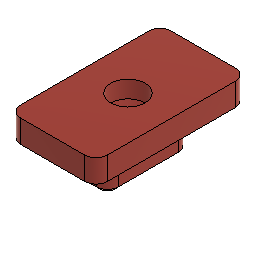
MEUBLE FAL_prod_BS (Autodesk Fusion 360 archive; units mm, degrees)
design "BLOCKOR_L36"
Autodesk Fusion 360 part; units mm, degrees
sketch "Sketch1" plane through (0, 0, 0) normal (0, 0, 1) x (1, 0, 0)
  line L0 (9, 18) -> (-9, 18)
  line L1 (-9, 18) -> (-9, -18)
  line L2 (-9, -18) -> (9, -18)
  line L3 (9, -18) -> (9, 18)
  line L4 (9, 18) -> (-9, -18) construction
  line L5 (-9, 18) -> (9, -18) construction
  dimension "d1" = 18
  dimension "d2" = 36
  constraint horizontal L0
  constraint perpendicular L0 L1
  constraint parallel L0 L2
  constraint parallel L1 L3
  constraint coincident L4 origin
  constraint coincident L5 origin
  measures "d1" distance of L0.start L0.end
  measures "d2" distance of L0.end L1.end
extrude "Extrude1" add sketch "Sketch1" along normal blind 16.5
sketch "Sketch2" plane through (0, 0, 16.5) normal (0, 0, 1) x (-1, 0, 0)
  line L0 (-9, 18) -> (-9, -18)
  line L1 (-9, -18) -> (9, -18)
  line L2 (9, -18) -> (9, 18)
  line L3 (9, 18) -> (-9, 18)
  line L4 (-19, -33) -> (19, -33)
  line L5 (19, -33) -> (19, 33)
  line L6 (19, 33) -> (-19, 33)
  line L7 (-19, 33) -> (-19, -33)
  line L8 (-19, -33) -> (19, 33) construction
  line L9 (19, -33) -> (-19, 33) construction
  dimension "d5" = 10
  dimension "d6" = 15
  constraint horizontal L4
  constraint perpendicular L4 L5
  constraint parallel L4 L6
  constraint parallel L5 L7
  constraint coincident L8 origin
  constraint coincident L9 origin
  measures "d5" distance of L2 L5
  measures "d6" distance of L1 L4
extrude "Extrude2" add sketch "Sketch2" along normal blind 10 contours L0 L1 L2 L3 | L4 L5 L6 L7
sketch "Sketch3" plane through (0, 0, 26.5) normal (0, 0, 1) x (-1, 0, 0)
  line L0 (-19, 33) -> (-19, -33)
  line L1 (-19, -33) -> (19, -33)
  line L2 (19, -33) -> (19, 33)
  line L3 (19, 33) -> (-19, 33)
  circle A0 centre (0, 0) radius 7.5
  dimension "d17" = 15
  constraint coincident A0.centre origin
  measures "d17" diameter of A0
extrude "Extrude3" cut sketch "Sketch3" against normal up to surface (10 mm away) contours A0
sketch "Sketch4" plane through (0, 0, 16.5) normal (0, 0, 1) x (-1, 0, 0)
  circle A0 centre (0, 0) radius 7.5
  constraint coincident A0.centre origin
hole "Hole2" at (0, 0, 16.5) direction (0, 0, -1) diameter 4.5 end through all countersink diameter 10 countersink angle 90
chamfer "Chamfer2" distance 2.5 angle 45 1 edges at (6.9925, 2.7121, 16.5)
fillet "Fillet1" radius 5 4 edges at (9, -18, 8.25) (-9, -18, 8.25) (9, 18, 8.25) (-9, 18, 8.25)
fillet "Fillet2" radius 5 4 edges at (-19, 33, 21.5) (19, 33, 21.5) (-19, -33, 21.5) (19, -33, 21.5)
chamfer "Chamfer1" distance 2 angle 45 8 edges at (0, 18, 0) (-7.5355, 16.5355, 0) (-9, 0, 0) (-7.5355, -16.5355, 0) (0, -18, 0) (7.5355, -16.5355, 0) (9, 0, 0) (7.5355, 16.5355, 0)

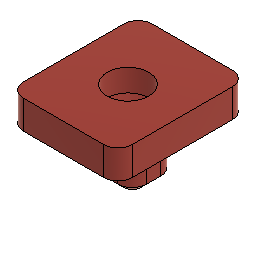
design "BLOCKOR_L15"
Autodesk Fusion 360 part; units mm, degrees
sketch "Sketch1" plane through (0, 0, 0) normal (0, 0, 1) x (1, 0, 0)
  line L0 (9, 7.5) -> (-9, 7.5)
  line L1 (-9, 7.5) -> (-9, -7.5)
  line L2 (-9, -7.5) -> (9, -7.5)
  line L3 (9, -7.5) -> (9, 7.5)
  line L4 (9, 7.5) -> (-9, -7.5) construction
  line L5 (-9, 7.5) -> (9, -7.5) construction
  dimension "d1" = 18
  dimension "d2" = 15
  constraint horizontal L0
  constraint perpendicular L0 L1
  constraint parallel L0 L2
  constraint parallel L1 L3
  constraint coincident L4 origin
  constraint coincident L5 origin
  measures "d1" distance of L0.start L0.end
  measures "d2" distance of L0.end L1.end
extrude "Extrude1" add sketch "Sketch1" along normal blind 16.5
sketch "Sketch2" plane through (0, 0, 16.5) normal (0, 0, 1) x (-1, 0, 0)
  line L0 (-9, 7.5) -> (-9, -7.5)
  line L1 (-9, -7.5) -> (9, -7.5)
  line L2 (9, -7.5) -> (9, 7.5)
  line L3 (9, 7.5) -> (-9, 7.5)
  line L4 (-19, -22.5) -> (19, -22.5)
  line L5 (19, -22.5) -> (19, 22.5)
  line L6 (19, 22.5) -> (-19, 22.5)
  line L7 (-19, 22.5) -> (-19, -22.5)
  line L8 (-19, -22.5) -> (19, 22.5) construction
  line L9 (19, -22.5) -> (-19, 22.5) construction
  dimension "d5" = 10
  dimension "d6" = 15
  constraint horizontal L4
  constraint perpendicular L4 L5
  constraint parallel L4 L6
  constraint parallel L5 L7
  constraint coincident L8 origin
  constraint coincident L9 origin
  measures "d5" distance of L2 L5
  measures "d6" distance of L1 L4
extrude "Extrude2" add sketch "Sketch2" along normal blind 10 contours L0 L1 L2 L3 | L4 L5 L6 L7
sketch "Sketch3" plane through (0, 0, 26.5) normal (0, 0, 1) x (-1, 0, 0)
  line L0 (-19, 22.5) -> (-19, -22.5)
  line L1 (-19, -22.5) -> (19, -22.5)
  line L2 (19, -22.5) -> (19, 22.5)
  line L3 (19, 22.5) -> (-19, 22.5)
  circle A0 centre (0, 0) radius 7.25
  dimension "d17" = 14.5
  constraint coincident A0.centre origin
  measures "d17" diameter of A0
fillet "Fillet1" radius 5 4 edges at (9, -7.5, 8.25) (-9, -7.5, 8.25) (9, 7.5, 8.25) (-9, 7.5, 8.25)
fillet "Fillet2" radius 5 4 edges at (-19, 22.5, 21.5) (19, 22.5, 21.5) (-19, -22.5, 21.5) (19, -22.5, 21.5)
chamfer "Chamfer1" distance 2 angle 45 8 edges at (0, 7.5, 0) (-7.5355, 6.0355, 0) (-9, 0, 0) (-7.5355, -6.0355, 0) (0, -7.5, 0) (7.5355, -6.0355, 0) (9, 0, 0) (7.5355, 6.0355, 0)
extrude "Extrude3" cut sketch "Sketch3" against normal up to surface (10 mm away) contours A0
sketch "Sketch4" plane through (0, 0, 16.5) normal (0, 0, 1) x (-1, 0, 0)
  circle A0 centre (0, 0) radius 7.25
  constraint coincident A0.centre origin
hole "Hole2" at (0, 0, 16.5) direction (0, 0, -1) diameter 4.5 end through all countersink diameter 10 countersink angle 90
chamfer "Chamfer2" distance 2.25 angle 45 1 edges at (6.7594, 2.6217, 16.5)

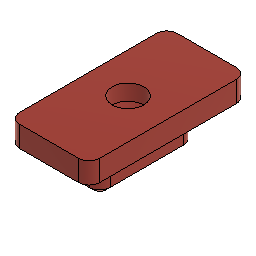
design "BLOCKOR_L45"
Autodesk Fusion 360 part; units mm, degrees
sketch "Sketch1" plane through (0, 0, 0) normal (0, 0, 1) x (1, 0, 0)
  line L0 (9, 22.5) -> (-9, 22.5)
  line L1 (-9, 22.5) -> (-9, -22.5)
  line L2 (-9, -22.5) -> (9, -22.5)
  line L3 (9, -22.5) -> (9, 22.5)
  line L4 (9, 22.5) -> (-9, -22.5) construction
  line L5 (-9, 22.5) -> (9, -22.5) construction
  dimension "d1" = 18
  dimension "d2" = 45
  constraint horizontal L0
  constraint perpendicular L0 L1
  constraint parallel L0 L2
  constraint parallel L1 L3
  constraint coincident L4 origin
  constraint coincident L5 origin
  measures "d1" distance of L0.start L0.end
  measures "d2" distance of L0.end L1.end
  measures "d5" distance of L0.start
  measures "d6" distance of L0.start
extrude "Extrude1" add sketch "Sketch1" along normal blind 16.5
sketch "Sketch2" plane through (0, 0, 16.5) normal (0, 0, 1) x (-1, 0, 0)
  line L0 (-9, 22.5) -> (-9, -22.5)
  line L1 (-9, -22.5) -> (9, -22.5)
  line L2 (9, -22.5) -> (9, 22.5)
  line L3 (9, 22.5) -> (-9, 22.5)
  line L4 (-19, -37.5) -> (19, -37.5)
  line L5 (19, -37.5) -> (19, 37.5)
  line L6 (19, 37.5) -> (-19, 37.5)
  line L7 (-19, 37.5) -> (-19, -37.5)
  line L8 (-19, -37.5) -> (19, 37.5) construction
  line L9 (19, -37.5) -> (-19, 37.5) construction
  dimension "d5" = 10
  dimension "d6" = 15
  constraint horizontal L4
  constraint perpendicular L4 L5
  constraint parallel L4 L6
  constraint parallel L5 L7
  constraint coincident L8 origin
  constraint coincident L9 origin
  measures "d5" distance of L2 L5
  measures "d6" distance of L1 L4
extrude "Extrude2" add sketch "Sketch2" along normal blind 10 contours L0 L1 L2 L3 | L4 L5 L6 L7
sketch "Sketch3" plane through (0, 0, 26.5) normal (0, 0, 1) x (-1, 0, 0)
  line L0 (-19, 37.5) -> (-19, -37.5)
  line L1 (-19, -37.5) -> (19, -37.5)
  line L2 (19, -37.5) -> (19, 37.5)
  line L3 (19, 37.5) -> (-19, 37.5)
  circle A0 centre (0, 0) radius 7.5
  dimension "d17" = 15
  constraint coincident A0.centre origin
  measures "d17" diameter of A0
extrude "Extrude3" cut sketch "Sketch3" against normal up to surface (10 mm away) contours A0
sketch "Sketch4" plane through (0, 0, 16.5) normal (0, 0, 1) x (-1, 0, 0)
  circle A0 centre (0, 0) radius 7.5
  constraint coincident A0.centre origin
hole "Hole2" at (0, 0, 16.5) direction (0, 0, -1) diameter 4.5 end through all countersink diameter 10 countersink angle 90
chamfer "Chamfer2" distance 2.5 angle 45 1 edges at (6.9925, 2.7121, 16.5)
fillet "Fillet1" radius 5 4 edges at (9, -22.5, 8.25) (-9, -22.5, 8.25) (9, 22.5, 8.25) (-9, 22.5, 8.25)
fillet "Fillet2" radius 5 4 edges at (-19, 37.5, 21.5) (19, 37.5, 21.5) (-19, -37.5, 21.5) (19, -37.5, 21.5)
chamfer "Chamfer1" distance 2 angle 45 8 edges at (0, 22.5, 0) (-7.5355, 21.0355, 0) (-9, 0, 0) (-7.5355, -21.0355, 0) (0, -22.5, 0) (7.5355, -21.0355, 0) (9, 0, 0) (7.5355, 21.0355, 0)

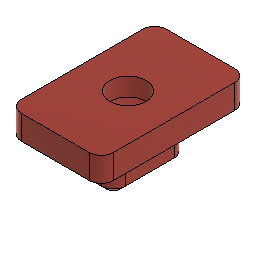
design "BLOCKOR_L30"
Autodesk Fusion 360 part; units mm, degrees
sketch "Sketch1" plane through (0, 0, 0) normal (0, 0, 1) x (1, 0, 0)
  line L0 (9, 15) -> (-9, 15)
  line L1 (-9, 15) -> (-9, -15)
  line L2 (-9, -15) -> (9, -15)
  line L3 (9, -15) -> (9, 15)
  line L4 (9, 15) -> (-9, -15) construction
  line L5 (-9, 15) -> (9, -15) construction
  dimension "d1" = 18
  dimension "d2" = 30
  constraint horizontal L0
  constraint perpendicular L0 L1
  constraint parallel L0 L2
  constraint parallel L1 L3
  constraint coincident L4 origin
  constraint coincident L5 origin
  measures "d1" distance of L0.start L0.end
  measures "d2" distance of L0.end L1.end
extrude "Extrude1" add sketch "Sketch1" along normal blind 16.5
sketch "Sketch2" plane through (0, 0, 16.5) normal (0, 0, 1) x (-1, 0, 0)
  line L0 (-9, 15) -> (-9, -15)
  line L1 (-9, -15) -> (9, -15)
  line L2 (9, -15) -> (9, 15)
  line L3 (9, 15) -> (-9, 15)
  line L4 (-19, -30) -> (19, -30)
  line L5 (19, -30) -> (19, 30)
  line L6 (19, 30) -> (-19, 30)
  line L7 (-19, 30) -> (-19, -30)
  line L8 (-19, -30) -> (19, 30) construction
  line L9 (19, -30) -> (-19, 30) construction
  dimension "d5" = 10
  dimension "d6" = 15
  constraint horizontal L4
  constraint perpendicular L4 L5
  constraint parallel L4 L6
  constraint parallel L5 L7
  constraint coincident L8 origin
  constraint coincident L9 origin
  measures "d5" distance of L2 L5
  measures "d6" distance of L1 L4
extrude "Extrude2" add sketch "Sketch2" along normal blind 10 contours L0 L1 L2 L3 | L4 L5 L6 L7
sketch "Sketch3" plane through (0, 0, 26.5) normal (0, 0, 1) x (-1, 0, 0)
  line L0 (-19, 30) -> (-19, -30)
  line L1 (-19, -30) -> (19, -30)
  line L2 (19, -30) -> (19, 30)
  line L3 (19, 30) -> (-19, 30)
  circle A0 centre (0, 0) radius 7.5
  dimension "d17" = 15
  constraint coincident A0.centre origin
  measures "d17" diameter of A0
fillet "Fillet1" radius 5 4 edges at (9, -15, 8.25) (-9, -15, 8.25) (9, 15, 8.25) (-9, 15, 8.25)
fillet "Fillet2" radius 5 4 edges at (-19, 30, 21.5) (19, 30, 21.5) (-19, -30, 21.5) (19, -30, 21.5)
chamfer "Chamfer1" distance 2 angle 45 8 edges at (0, 15, 0) (-7.5355, 13.5355, 0) (-9, 0, 0) (-7.5355, -13.5355, 0) (0, -15, 0) (7.5355, -13.5355, 0) (9, 0, 0) (7.5355, 13.5355, 0)
extrude "Extrude3" cut sketch "Sketch3" against normal up to surface (10 mm away) contours A0
sketch "Sketch4" plane through (0, 0, 16.5) normal (0, 0, 1) x (-1, 0, 0)
  circle A0 centre (0, 0) radius 7.5
  constraint coincident A0.centre origin
hole "Hole2" at (0, 0, 16.5) direction (0, 0, -1) diameter 4.5 end through all countersink diameter 10 countersink angle 90
chamfer "Chamfer2" distance 2.5 angle 45 1 edges at (6.9925, 2.7121, 16.5)

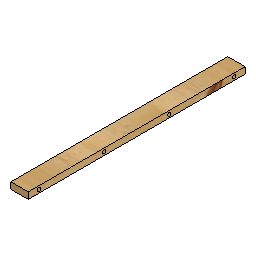
design "DEMI-ETAGERE"
Autodesk Fusion 360 part; units mm, degrees
sketch "Sketch1" plane through (0, 0, 0) normal (1, 0, 0) x (0, 1, 0)
  line L0 (250, -7.5) -> (-250, -7.5)
  line L1 (-250, -7.5) -> (-250, 7.5)
  line L2 (-250, 7.5) -> (250, 7.5)
  line L3 (250, 7.5) -> (250, -7.5)
  line L4 (250, -7.5) -> (-250, 7.5) construction
  line L5 (-250, -7.5) -> (250, 7.5) construction
  dimension "d1" = 15
  dimension "d2" = 500
  constraint perpendicular L0 L1
  constraint parallel L0 L2
  constraint parallel L1 L3
  constraint horizontal L0
  constraint coincident L4 origin
  constraint coincident L5 origin
  measures "d1" distance of L0.end L1.end
  measures "d2" distance of L1.end L2.end
extrude "Extrude1" add sketch "Sketch1" along normal blind 40
sketch "Sketch2" plane through (40, 0, 0) normal (1, 0, 0) x (0, 1, 0)
  line L0 (250, 7.5) -> (-250, 7.5)
  line L1 (-250, 7.5) -> (-250, -7.5)
  line L2 (-250, -7.5) -> (250, -7.5)
  line L3 (250, -7.5) -> (250, 7.5)
  line L4 (0, 7.5) -> (0, -7.5) construction
  line L5 (0, 0) -> (-75, 0) construction
  line L6 (-75, 0) -> (-225, 0) construction
  point P0 (-75, 0)
  point P1 (-225, 0)
  dimension "d5" = 75
  dimension "d6" = 225
  constraint midpoint L0 L4.start
  constraint midpoint L2 L4.end
  constraint coincident L5.start origin
  constraint perpendicular L4 L5
  constraint parallel L0 L6
  constraint coincident P0 L5.end
  constraint coincident P1 L6.end
  measures "d5" distance of L5.start L5.end
  measures "d6" distance of L5.start P1
hole "Hole1" at (40, -75, 0) at (40, -225, 0) direction (-1, 0, 0) diameter 8 depth 30 tip angle 118
mirror "Mirror1" about plane through (0, 0, 0) normal (0, 1, 0) of "Hole1"
